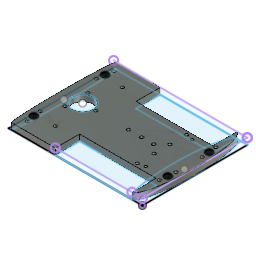
chassis (Autodesk Fusion 360 design; units mm, degrees)
Autodesk Fusion 360 part; units mm, degrees
sketch "Esquisse1" plane through (0, 0, 0) normal (0, 0, 1) x (1, 0, 0)
  line L0 (0, 0) -> (-127.5, 0)
  line L1 (-127.5, 0) -> (-127.5, 100)
  line L2 (-127.5, 100) -> (0, 100)
  line L3 (0, 100) -> (0, 0)
  ellipse E0 centre (-10, 50) end of major axis (0, 50) minor radius 50
  line L4 (-20, 50) -> (0, 50)
  line L5 (-10, 0) -> (-10, 100)
  ellipse E1 centre (-125, 50) end of major axis (-127.5, 50) minor radius 50
  line L6 (-122.5, 50) -> (-127.5, 50)
  line L7 (-125, 100) -> (-125, 0)
  line L8 (-10, 100) -> (-83, 100)
  line L9 (-83, 100) -> (-83, 77)
  line L10 (-83, 77) -> (-10, 77)
  line L11 (-10, 77) -> (-10, 100)
  line L12 (-10, 0) -> (-83, 0)
  line L13 (-83, 0) -> (-83, 23)
  line L14 (-83, 23) -> (-10, 23)
  line L15 (-10, 23) -> (-10, 0)
  dimension "d1" = 127.5
  dimension "d2" = 73
  dimension "d3" = 23
  dimension "d4" = 73
  dimension "d5" = 23
  constraint horizontal L0
  constraint vertical L1
  constraint horizontal L2
  constraint vertical L3
  constraint coincident L0.start L3.end
  constraint perpendicular L3 L4
  constraint coincident E0 L4.start
  constraint coincident E0 L4.end
  constraint coincident E0 L5.start
  constraint coincident E0 L5.end
  constraint perpendicular L1 L6
  constraint coincident E1 L6.start
  constraint coincident E1 L6.end
  constraint coincident E1 L7.start
  constraint coincident E1 L7.end
  constraint horizontal L8
  constraint vertical L9
  constraint horizontal L10
  constraint vertical L11
  constraint horizontal L12
  constraint vertical L13
  constraint horizontal L14
  constraint vertical L15
  measures "d1" distance of L0.start L0.end
  measures "d2" distance of L5.end L8.end
  measures "d3" distance of L5.end L10.end
  measures "d4" distance of L5.start L12.end
  measures "d5" distance of L5.start L14.end
extrude "Extrusion1" add sketch "Esquisse1" along normal blind 6 contours E0 L4 L5 L15 | E0 L4 L5 L11 | L0 L2 E0 E1 L9 L10 L13 L14 | E0 L4 L5 L14 | E0 L4 L5 L10 | E1 L6 L7 | E1 L6 L7 | E1 L6 L7 | E1 L6 L7
sketch "Esquisse2" plane through (0, 0, 6) normal (0, 0, 1) x (-1, 0, 0)
  line L0 (83, 0) -> (83, -23)
  line L1 (83, -23) -> (10, -23)
  line L2 (10, -23) -> (10, 0)
  ellipse E0 centre (10, -50) end of major axis (10, -100) minor radius 10 (10, 0) -> (10, -100) ccw
  line L3 (10, -100) -> (10, -77)
  line L4 (10, -77) -> (83, -77)
  line L5 (83, -77) -> (83, -100)
  line L6 (83, -100) -> (125, -100)
  ellipse E1 centre (125, -50) end of major axis (125, 0) minor radius 2.5 (125, -100) -> (125, 0) ccw
  line L7 (125, 0) -> (83, 0)
  circle A0 centre (107, -50) radius 10
  circle A1 centre (119.6, -16) radius 3
  circle A2 centre (119.6, -84) radius 3
  line L8 (0, -100) -> (0, 0)
  line L9 (127.5, -100) -> (0, -100)
  circle A3 centre (6, -30.25) radius 3
  line L10 (10, 0) -> (83, 0)
  circle A4 centre (6, -69.75) radius 3
  dimension "d8" = 20
  dimension "d9" = 6
  dimension "d10" = 16
  dimension "d11" = 119.6
  dimension "d12" = 6
  dimension "d13" = 119.6
  dimension "d14" = 16
  dimension "d15" = 6
  dimension "d16" = 30.25
  dimension "d17" = 6
  dimension "d18" = 6
  dimension "d19" = 6
  dimension "d20" = 30.25
  dimension "d49" = 107
  measures "d8" diameter of A0
  measures "d9" diameter of A1
  measures "d10" distance of L7 A1.centre
  measures "d11" horizontal distance of L8.end A1.centre
  measures "d12" diameter of A2
  measures "d13" distance of A2.centre L8
  measures "d14" distance of A2.centre L9
  measures "d15" diameter of A3
  measures "d16" distance of A3.centre L10
  measures "d17" distance of L8 A3.centre
  measures "d18" diameter of A4
  measures "d19" distance of L8 A4.centre
  measures "d20" distance of L9 A4.centre
  measures "d49" distance of A0.centre L8
extrude "Extrusion2" cut sketch "Esquisse2" against normal blind 7 contours A0 | A1 | A2 | A3 | A4
sketch "Esquisse3" plane through (0, 0, 6) normal (0, 0, 1) x (-1, 0, 0)
  circle A0 centre (119.6, -16) radius 3
  circle A1 centre (107, -50) radius 10
  circle A2 centre (6, -30.25) radius 3
  circle A3 centre (119.6, -84) radius 3
  circle A4 centre (6, -69.75) radius 3
  line L0 (83, 0) -> (83, -23)
  line L1 (83, -23) -> (10, -23)
  line L2 (10, -23) -> (10, 0)
  ellipse E0 centre (10, -50) end of major axis (10, -100) minor radius 10 (10, 0) -> (10, -100) ccw
  line L3 (10, -100) -> (10, -77)
  line L4 (10, -77) -> (83, -77)
  line L5 (83, -77) -> (83, -100)
  line L6 (83, -100) -> (125, -100)
  ellipse E1 centre (125, -50) end of major axis (125, 0) minor radius 2.5 (125, -100) -> (125, 0) ccw
  line L7 (125, 0) -> (83, 0)
  circle A5 centre (39.3, -49.9) radius 1.5
  line L8 (0, -100) -> (0, 0)
  line L9 (10, 0) -> (83, 0)
  circle A6 centre (50.8, -49.9) radius 1.5
  circle A7 centre (63.3, -49.9) radius 1.5
  line L10 (0, 0) -> (127.5, 0)
  circle A8 centre (31.3, -26.5) radius 1.5
  circle A9 centre (31.3, -42.5) radius 1.5
  circle A10 centre (101.15, -18) radius 1.5
  circle A11 centre (112.9372, -39) radius 1.5
  circle A12 centre (94.5, -50) radius 1.5
  circle A13 centre (118.55, -8.8) radius 1.5
  circle A14 centre (120.65, -23.2) radius 1.5
  circle A15 centre (24.6, -27.8) radius 1.25
  circle A16 centre (7, -23) radius 1.5
  circle A17 centre (5.5, -37.5) radius 1.5
  point P0 (107, -50)
  dimension "d23" = 3
  dimension "d24" = 39.3
  dimension "d25" = 49.9
  dimension "d26" = 3
  dimension "d27" = 49.9
  dimension "d28" = 50.8
  dimension "d29" = 3
  dimension "d30" = 63.3
  dimension "d31" = 49.9
  dimension "d32" = 3
  dimension "d33" = 26.5
  dimension "d34" = 31.3
  dimension "d35" = 3
  dimension "d36" = 31.3
  dimension "d37" = 42.5
  dimension "d38" = 3
  dimension "d39" = 18
  dimension "d40" = 101.15
  dimension "d41" = 3
  dimension "d44" = 3
  dimension "d45" = 50
  dimension "d46" = 94.5
  dimension "d51" = 12.5
  dimension "d52" = 39
  dimension "d53" = 3
  dimension "d54" = 8.8
  dimension "d55" = 118.55
  dimension "d56" = 3
  dimension "d57" = 120.65
  dimension "d58" = 23.2
  dimension "d59" = 2.5
  dimension "d60" = 27.8
  dimension "d61" = 24.6
  dimension "d62" = 3
  dimension "d63" = 23
  dimension "d64" = 7
  dimension "d65" = 3
  dimension "d66" = 5.5
  dimension "d67" = 37.5
  measures "d23" diameter of A5
  measures "d24" distance of A5.centre L8
  measures "d25" distance of A5.centre L9
  measures "d26" diameter of A6
  measures "d27" distance of L9 A6.centre
  measures "d28" distance of L8 A6.centre
  measures "d29" diameter of A7
  measures "d30" distance of L8 A7.centre
  measures "d31" distance of A7.centre L10
  measures "d32" diameter of A8
  measures "d33" distance of L9 A8.centre
  measures "d34" distance of L8 A8.centre
  measures "d35" diameter of A9
  measures "d36" distance of L8 A9.centre
  measures "d37" distance of L10 A9.centre
  measures "d38" diameter of A10
  measures "d39" distance of L9 A10.centre
  measures "d40" distance of L8 A10.centre
  measures "d41" diameter of A11
  measures "d44" diameter of A12
  measures "d45" distance of L9 A12.centre
  measures "d46" distance of L8 A12.centre
  measures "d51" distance of A11.centre P0
  measures "d52" distance of L10 A11.centre
  measures "d53" diameter of A13
  measures "d54" distance of L10 A13.centre
  measures "d55" distance of L8 A13.centre
  measures "d56" diameter of A14
  measures "d57" distance of L8 A14.centre
  measures "d58" distance of L10 A14.centre
  measures "d59" diameter of A15
  measures "d60" distance of L10 A15.centre
  measures "d61" distance of L8 A15.centre
  measures "d62" diameter of A16
  measures "d63" distance of L10 A16.centre
  measures "d64" distance of L8 A16.centre
  measures "d65" diameter of A17
  measures "d66" distance of L8 A17.centre
  measures "d67" distance of L10 A17.centre
extrude "Extrusion3" cut sketch "Esquisse3" against normal blind 6 contours A5 | A6 | A7 | A8 | A9 | A10 | A11 | A12 | A13 | A14 | A15 | A16 | A17
ref_plane "Plan de construction1" through (-104, 50, 3) normal (0, 1, 0) x (-1, 0, 0)
mirror "Symétrie miroir1" about plane through (-104, 50, 3) normal (0, 1, 0) of "Extrusion3"
